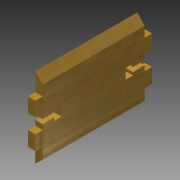
# Autodesk Inventor part: lateralnova
Saved by Autodesk Inventor 2014 (Build 180170000, 170)
## iProperties
Created: 2015-11-06
Part Number: lateralnova
Material: Generic
Document SubType Name: Modeling
Designer: Gabriel
Density: 1 g/cm^3
Appearance: Default
Author: Gabriel
Autodesk Inventor part; units mm, degrees
ref_plane "YZ Plane" through (0, 0, 0) normal (1, 0, 0) x (0, 1, 0)
ref_plane "XZ Plane" through (0, 0, 0) normal (0, 1, 0) x (-1, 0, 0)
ref_plane "XY Plane" through (0, 0, 0) normal (0, 0, 1) x (1, 0, 0)
sketch "Sketch2" plane through (0, 0, 0) normal (0, 1, 0) x (-1, 0, 0)
  line L0 (0, 0) -> (5, 0)
  line L1 (5, 0) -> (5, -54.829)
  line L2 (5, -54.829) -> (0, -54.829)
  line L3 (0, -54.829) -> (0, 0)
  dimension "d0" = 5
  dimension "d1" = 54.829
  constraints: 8 end point, 2 parallel, 1 horizontal, 1 perpendicular
  measures "d0" distance of L1.end L2.end
  measures "d1" distance of L0.end L1.end
extrude "Extrusion1" add sketch "Sketch2" along normal blind 70
sketch "Sketch4" plane through (0, 70, 0) normal (0, 1, 0) x (1, 0, 0)
  line L0 (0, 0) -> (0, 54.829)
  line L1 (0, 54.829) -> (-5, 54.829)
  line L2 (-5, 54.829) -> (-5, 0)
  line L3 (-5, 0) -> (0, 0)
  line L4 (-5, 0) -> (-5, 12.5)
  line L5 (-5, 12.5) -> (0, 12.5)
  line L6 (-5, 12.5) -> (-5, 22.5)
  line L7 (-5, 22.5) -> (0, 22.5)
  line L8 (0, 22.5) -> (0, 32.5)
  line L9 (0, 32.5) -> (-5, 32.5)
  line L10 (-5, 32.5) -> (-5, 42.5)
  line L11 (-5, 42.5) -> (0, 42.5)
  dimension "d8" = 12.5
  dimension "d9" = 10
  dimension "d10" = 10
  dimension "d11" = 10
  constraints: 24 end point, 8 point on line, 5 perpendicular, 2 parallel
  measures "d8" distance of L2.end L4.end
  measures "d9" distance of L4.end L6.end
  measures "d10" distance of L7.end L8.end
  measures "d11" distance of L9.end L10.end
extrude "Extrusion2" add sketch "Sketch4" along normal blind 5 contours L5 L2 L7 L0 | L9 L2 L11 L0
sketch "Sketch5" plane through (0, 0, 0) normal (0, -1, 0) x (1, 0, 0)
  line L0 (-5, 0) -> (0, 0)
  line L1 (0, 0) -> (0, -54.829)
  line L2 (-5, 0) -> (-5, -12.5)
  line L3 (-5, -12.5) -> (0, -12.5)
  line L4 (-5, -12.5) -> (-5, -22.5)
  line L5 (-5, -22.5) -> (0, -22.5)
  line L6 (-5, -22.5) -> (-5, -32.5)
  line L7 (-5, -32.5) -> (0, -32.5)
  line L8 (-5, -32.5) -> (-5, -42.5)
  line L9 (-5, -42.5) -> (0, -42.5)
  line L10 (-5, -42.5) -> (-5, -54.829)
  line L11 (0, -54.829) -> (-5, -54.829)
  line L12 (0, 0) -> (0, -5.504)
  line L13 (0, -5.504) -> (-5, 0)
  line L14 (0, -54.829) -> (0, -50.141)
  line L15 (0, -50.141) -> (-5, -54.829)
  dimension "d20" = 10
  dimension "d21" = 10
  dimension "d22" = 10
  dimension "d23" = 12.5
  dimension "d24" = 54.829
  dimension "d25" = 12.329
  dimension "d28" = 5.504
  dimension "d29" = 4.688
  constraints: 32 end point, 9 perpendicular, 6 point on line, 1 parallel
  measures "d20" distance of L2.end L4.end
  measures "d21" distance of L4.end L6.end
  measures "d22" distance of L6.end L8.end
  measures "d23" distance between parallel lines of L3 L0
  measures "d24" distance between parallel lines of L11 L0
  measures "d25" distance between parallel lines of L11 L9
  measures "d28" distance of L0.end L12.end
  measures "d29" distance of L1.end L14.end
extrude "Extrusion3" add sketch "Sketch5" along normal blind 5 contours L3 L1 L5 L4 | L7 L1 L9 L8
extrude "Extrusion4" cut sketch "Sketch5" against normal blind 70 contours L0 L1 L13 | L15 L1 L11
sketch "Sketch6" plane through (-5, 70, -12.5) normal (-1, 0, 0) x (0, 0, 1)
  line L0 (-13.5, -70) -> (-15, -70)
  line L1 (-15, -70) -> (-13.5, -70)
  line L2 (-13.5, -70) -> (-15, -70)
  line L3 (-15, -70) -> (-16.5, -70)
  line L4 (-16.5, -70) -> (-15, -70)
  line L5 (-13.5, -70) -> (-13.5, -62)
  line L6 (-13.5, -62) -> (-11.5, -62)
  line L7 (-11.5, -62) -> (-11.5, -57)
  line L8 (-13.5, -70) -> (-16.5, -70)
  line L9 (-16.5, -70) -> (-16.5, -62)
  line L10 (-16.5, -62) -> (-18.5, -62)
  line L11 (-18.5, -62) -> (-18.5, -57)
  line L12 (-18.5, -57) -> (-11.5, -57)
  line L13 (-13.5, 0) -> (-15, 0)
  line L14 (-15, 0) -> (-13.5, 0)
  line L15 (-13.5, 0) -> (-15, 0)
  line L16 (-15, 0) -> (-16.5, 0)
  line L17 (-16.5, 0) -> (-15, 0)
  line L18 (-13.5, 0) -> (-13.5, -8)
  line L19 (-13.5, -8) -> (-11.5, -8)
  line L20 (-11.5, -8) -> (-11.5, -13)
  line L21 (-13.5, 0) -> (-16.5, 0)
  line L22 (-16.5, 0) -> (-16.5, -8)
  line L23 (-16.5, -8) -> (-18.5, -8)
  line L24 (-18.5, -8) -> (-18.5, -13)
  line L25 (-18.5, -13) -> (-11.5, -13)
  point P0 (12.5, -70)
  dimension "d35" = 1.5
  dimension "d36" = 8
  dimension "d37" = 2
  dimension "d38" = 5
  dimension "d39" = 2
  constraints: 52 end point, 6 perpendicular, 4 collinear
  measures "d35" distance of L0.end L3.end
  measures "d36" distance of L0.start L5.end
  measures "d37" distance of L5.end L6.end
  measures "d38" distance of L6.end L7.end
  measures "d39" distance of L9.end L10.end
extrude "Extrusion5" cut sketch "Sketch6" against normal blind 5
body "Solid1"
